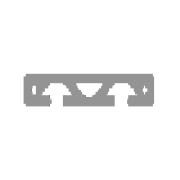
# Autodesk Inventor part: 10-081
Saved by Autodesk Inventor 2022 (Build 260153000, 153)
## iProperties
Created: 2021-12-28
Part Number: 10-081
Material: Generico
Document SubType Name: Modeling
Designer: matte
Standards Organization: 40 series
Language: it-IT
Size Designation: 10-081
Categories: <MemberInstance><Categories><Category DisplayName="Forme strutturali" InternalName="089c4875-fa83-4c05-b084-43b9cc11f5ed" Mnemonic="GRDR"><CategoryParameter DisplayName="Massa per unità di lunghezza" InternalName="0bb95a10-148f-4027-a459-38d7b056702a" Mnemonic="shpmass"/><CategoryParameter DisplayName="Area sezione" InternalName="1ff91680-64b0-4202-b9a3-7fd3f94bba3b" Mnemonic="secarea"/><CategoryParameter DisplayName="Raggio di girazione (x)" InternalName="25778675-03e9-40c1-b6a8-4a9ed693320d" Mnemonic="gyrradx"/><CategoryParameter DisplayName="Modulo di rigidità torsionale" InternalName="26c1ec35-5026-4c63-ad0a-751cf684a536" Mnemonic="torrigmod"/><CategoryParameter DisplayName="Distanza del baricentro X-X" InternalName="26c9bdb8-9c79-4b4f-a92e-8e197583c9c4" Mnemonic="grcendistX"/><CategoryParameter DisplayName="ID membro precedente" InternalName="340afe4f-75d7-48d3-ab7d-943f3c3da468" Mnemonic="LegacyMemberID"/><CategoryParameter DisplayName="Lunghezza base" InternalName="42e34263-8f20-4d0e-ad48-bf1385b87c24" Mnemonic="shplen"/><CategoryParameter DisplayName="Momento di inerzia (y)" InternalName="4b9f58ea-bced-460e-81ea-3d29ca5a49e3" Mnemonic="inermomy"/><CategoryParameter DisplayName="Momento di inerzia (x)" InternalName="4cd780bc-73d7-43ac-917a-579e5cbd684d" Mnemonic="inermomx"/><CategoryParameter DisplayName="Punto di base personalizzato" InternalName="4f1d1b73-316d-484b-a3df-9cbabb16eb77" Mnemonic="shpBasePoint"/><CategoryParameter DisplayName="Altezza forma" InternalName="50274e7d-5ac0-4796-92cb-c59e54983c67" Mnemonic="shpheig"/><CategoryParameter DisplayName="Modulo sezione (y)" InternalName="59eaa5e9-d227-48dc-b6c1-6920f96e0f95" Mnemonic="secmody"/><CategoryParameter DisplayName="Designazione sezione" InternalName="5a64d034-428d-49c8-ba32-7619764de20f" Mnemonic="shpdes"/><CategoryParameter DisplayName="Modulo sezione (x)" InternalName="72cfad18-cf51-4ed4-aaa7-c6b224f8419f" Mnemonic="secmodx"/><CategoryParameter DisplayName="Modulo di sezione torsionale" InternalName="7c55a8dc-8844-49f9-a867-cc677b30ec9a" Mnemonic="torsecmod"/><CategoryParameter DisplayName="Larghezza forma" InternalName="7c717d54-a18f-4666-b4d4-573cce22c62c" Mnemonic="shpwdth"/><CategoryParameter DisplayName="Spessore seconda forma" InternalName="9251a8e1-85fd-4e47-af99-afdb762317d9" Mnemonic="shpthick2"/><CategoryParameter DisplayName="Guarnizione piatta creata" InternalName="9c666724-f362-4ea7-ac62-f6a007de5c69" Mnemonic="shpFGAuto"/><CategoryParameter DisplayName="Distanza del baricentro Y-Y" InternalName="bcc4fb17-7af4-436a-8f8c-d0aa3b0248c5" Mnemonic="grcendistY"/><CategoryParameter DisplayName="Raggio di girazione (y)" InternalName="bfa18ebe-1636-4dbe-8d42-b263e0b73184" Mnemonic="gyrrady"/><CategoryParameter DisplayName="Spessore forma" InternalName="d109cf76-8eb4-42fc-9800-4409734adc67" Mnemonic="shpthick"/><CategoryParameter DisplayName="Coefficiente di spostamento taglio" InternalName="de4c90c6-aaa8-468f-a335-6737b311b5d3" Mnemonic="shdispc"/><Category DisplayName="Altro" InternalName="f02205ff-2390-476f-921c-0b3185f88e84" Mnemonic="OTHSHP"><CategoryParameter DisplayName="Momento di inerzia (y)" InternalName="044c654e-f649-48ac-84cc-650a29ae31ca" Mnemonic="inermomy"/><CategoryParameter DisplayName="Spessore forma" InternalName="12b1a788-9233-48fd-a933-2df8ff42b15f" Mnemonic="shpthick"/><CategoryParameter DisplayName="Massa per unità di lunghezza" InternalName="2fd289d6-9394-4d2d-97e6-6659d7d4551d" Mnemonic="shpmass"/><CategoryParameter DisplayName="Raggio di girazione (y)" InternalName="743e1dfe-1bba-408b-b985-cf752b207386" Mnemonic="gyrrady"/><CategoryParameter DisplayName="Modulo sezione (y)" InternalName="88b8bff9-a616-4028-93d5-ed4f79680d13" Mnemonic="secmody"/><CategoryParameter DisplayName="Area sezione" InternalName="c46ecdf8-b6eb-4db9-8b25-30258930c1e3" Mnemonic="secarea"/><CategoryParameter DisplayName="Modulo sezione (x)" InternalName="cac70804-9d39-43bb-be17-56ea1f39a6c2" Mnemonic="secmodx"/><CategoryParameter DisplayName="Momento di inerzia (x)" InternalName="ec6737bc-264f-43ed-b0bd-f6d410c2718d" Mnemonic="inermomx"/><CategoryParameter DisplayName="Raggio di girazione (x)" InternalName="ee72c61e-565e-4fd6-b448-66e1e1abcb7e" Mnemonic="gyrradx"/></Category></Category><Category DisplayName="TipoDati" InternalName="23b78d0f-2648-40c6-8793-ca6db495c9e8" Mnemonic="DATATYPE"><CategoryParameter DisplayName="NomeVisualizzazione" InternalName="05415f3d-3907-474b-a020-eb9d644f4cf3" Mnemonic="DISPLAYNAME"/><CategoryParameter DisplayName="Norme" InternalName="0c0a119c-1e12-4c84-803f-101930972f5e" Mnemonic="STANDARD"/><CategoryParameter DisplayName="Descrizione" InternalName="13903e3d-64b1-4950-80da-f627842ea37f" Mnemonic="DESCRIPTION"/><CategoryParameter DisplayName="Designazione" InternalName="2675968c-4ce5-49e0-a4f5-552d29089031" Mnemonic="DESIGNATION"/><CategoryParameter DisplayName="Riga di default" InternalName="2af9ec52-faaa-4026-b378-f9fa4afca842" Mnemonic="DEFAULTROW"/><CategoryParameter DisplayName="Nome cartella" InternalName="3f06958e-8713-4116-9be7-ed6184ecc97b" Mnemonic="FOLDERNAME"/><CategoryParameter DisplayName="Guid revisione" InternalName="45a75005-10b1-4dfc-8d6d-dfe629f0b93c" Mnemonic="REVISIONGUID"/><CategoryParameter DisplayName="NomeFile" InternalName="8b46a4cc-9585-4fed-90c3-899f57e09a73" Mnemonic="FILENAME"/><CategoryParameter DisplayName="SocietàNorme" InternalName="8f5914e1-4693-403f-8ab5-d37768198c9d" Mnemonic="STDSORG"/><CategoryParameter DisplayName="Versione famiglia" InternalName="914462f6-6e19-4b14-ba84-155b9680b1d0" Mnemonic="FAMILYREVISION"/><CategoryParameter DisplayName="Revisione norme" InternalName="91d5a463-65c2-4fde-b823-3b7fea5e8e17" Mnemonic="STANDARDREVISION"/><CategoryParameter DisplayName="Revisione membro" InternalName="a65d44b9-392f-4f4f-857b-e4b3d54996fe" Mnemonic="MEMBERREVISION"/><CategoryParameter DisplayName="FormatoPianoRitaglio" InternalName="bc51e27b-3422-4e78-93ef-cec197ddf230" Mnemonic="CLIPFORMAT"/><CategoryParameter DisplayName="Produttore" InternalName="cd6c7a72-a28a-4e50-99a9-2c7f4e13e5ad" Mnemonic="MANUFACTURER"/><CategoryParameter DisplayName="NomeInterno" InternalName="cf1d0246-76d9-4b4a-8305-fa0409afb5c1" Mnemonic="INTERNALNAME"/><CategoryParameter DisplayName="Èmetrico" InternalName="e2385c5b-1ea4-4823-96a8-8de651266ec3" Mnemonic="ISMETRIC"/><Category DisplayName="Parte" InternalName="c0e0b642-3bcb-4cc8-9e80-f96d35c4afa4" Mnemonic="PART"><CategoryParameter DisplayName="Numero parte" InternalName="016b6077-bfbe-49bd-92c9-d8d59c39c941" Mnemonic="PARTNUMBER"/><CategoryParameter DisplayName="Numero di magazzino" InternalName="4dba7c1c-e26c-444e-836c-b08b433409a8" Mnemonic="STOCKNUMBER"/><CategoryParameter DisplayName="Chiave materiale" InternalName="5c9a8adb-dd2b-4535-b97f-0a94a95fe41f" Mnemonic="MATERIALKEY"/><CategoryParameter DisplayName="Materiale" InternalName="818a152a-d3c3-49ca-80ee-df7d91421b8e" Mnemonic="MATERIAL"/></Category></Category></Categories><FamilyTemplate Id="10-081"><FamilyTemplateParameters><FamilyTemplateParameter ObjectType="kModelParameterObject" ValueType="xs:double" Id="12" ObjectReferenceKey="d8"/><FamilyTemplateParameter ObjectType="kPartComponentDefinitionObject" ValueType="xs:string" Id="23" SubObjectId="Material"/><FamilyTemplateParameter ObjectType="kPropertyObject" ValueType="xs:string" Id="26" ObjectReferenceKey="{32853F0F-3444-11d1-9E93-0060B03C1CA6}" SubObjectId="5"/><FamilyTemplateParameter ObjectType="kPropertyObject" ValueType="xs:string" Id="27" ObjectReferenceKey="{32853F0F-3444-11d1-9E93-0060B03C1CA6}" SubObjectId="52"/></FamilyTemplateParameters></FamilyTemplate><CategoryParameterMap><ParamToTemplateMap><ParamToTemplate CategoryParameter="//CategoryParameter[@InternalName='cf1d0246-76d9-4b4a-8305-fa0409afb5c1']" ConstantValue="b43aa390-bf45-4392-bb08-a6c8910b2740"/><ParamToTemplate CategoryParameter="//CategoryParameter[@InternalName='45a75005-10b1-4dfc-8d6d-dfe629f0b93c']" ConstantValue="b3b43e47-2cae-4de0-b985-6c6fa3d76176"/><ParamToTemplate CategoryParameter="//CategoryParameter[@InternalName='3f06958e-8713-4116-9be7-ed6184ecc97b']" ConstantValue="10-081"/><ParamToTemplate CategoryParameter="//CategoryParameter[@InternalName='8f5914e1-4693-403f-8ab5-d37768198c9d']" ConstantValue="40 series"/><ParamToTemplate CategoryParameter="//CategoryParameter[@InternalName='0c0a119c-1e12-4c84-803f-101930972f5e']" TemplateParameter="18"/><ParamToTemplate CategoryParameter="//CategoryParameter[@InternalName='91d5a463-65c2-4fde-b823-3b7fea5e8e17']" TemplateParameter="19"/><ParamToTemplate CategoryParameter="//CategoryParameter[@InternalName='cd6c7a72-a28a-4e50-99a9-2c7f4e13e5ad']" TemplateParameter="20"/><ParamToTemplate CategoryParameter="//CategoryParameter[@InternalName='13903e3d-64b1-4950-80da-f627842ea37f']" TemplateParameter="22"/><ParamToTemplate CategoryParameter="//CategoryParameter[@InternalName='05415f3d-3907-474b-a020-eb9d644f4cf3']" ConstantValue="10-081"/><ParamToTemplate CategoryParameter="//CategoryParameter[@InternalName='914462f6-6e19-4b14-ba84-155b9680b1d0']" ConstantValue="11"/><ParamToTemplate CategoryParameter="//CategoryParameter[@InternalName='bc51e27b-3422-4e78-93ef-cec197ddf230']" ConstantValue="CF_INVENTOR.STDPARTS"/><ParamToTemplate CategoryParameter="//CategoryParameter[@InternalName='e2385c5b-1ea4-4823-96a8-8de651266ec3']" ConstantValue="true"/><ParamToTemplate CategoryParameter="//CategoryParameter[@InternalName='2af9ec52-faaa-4026-b378-f9fa4afca842']" ConstantValue="1"/><ParamToTemplate CategoryParameter="//CategoryParameter[@InternalName='9c666724-f362-4ea7-ac62-f6a007de5c69']" ConstantValue="1"/><ParamToTemplate CategoryParameter="//CategoryParameter[@InternalName='8b46a4cc-9585-4fed-90c3-899f57e09a73']" ConstantValue="10-081"/><ParamToTemplate CategoryParameter="//CategoryParameter[@InternalName='a65d44b9-392f-4f4f-857b-e4b3d54996fe']" ConstantValue="bb38fb4f-2023-4888-b702-42cbc433ea70"/><ParamToTemplate CategoryParameter="//CategoryParameter[@InternalName='a65d44b9-392f-4f4f-857b-e4b3d54996fe']" ConstantValue="bb38fb4f-2023-4888-b702-42cbc433ea70"/><ParamToTemplate CategoryParameter="//CategoryParameter[@InternalName='2675968c-4ce5-49e0-a4f5-552d29089031']" TemplateParameter="27"/><ParamToTemplate CategoryParameter="//CategoryParameter[@InternalName='818a152a-d3c3-49ca-80ee-df7d91421b8e']" TemplateParameter="23"/><ParamToTemplate CategoryParameter="//CategoryParameter[@InternalName='016b6077-bfbe-49bd-92c9-d8d59c39c941']" TemplateParameter="26"/><ParamToTemplate CategoryParameter="//CategoryParameter[@InternalName='42e34263-8f20-4d0e-ad48-bf1385b87c24']" TemplateParameter="12"/></ParamToTemplateMap></CategoryParameterMap></MemberInstance>
Density: 1 g/cm^3
Appearance: Default
MXEDIT: true
G_L: 240,000 mm
IsCustomPart: 1
Author: matte
Autodesk Inventor part; units mm, degrees
ref_plane "YZ Plane" through (0, 0, 0) normal (1, 0, 0) x (0, 1, 0)
ref_plane "Start Plane" through (0, 0, 0) normal (0, 1, 0) x (-1, 0, 0)
ref_plane "End Plane" through (0, 240, 0) normal (0, 1, 0) x (-1, 0, 0)
sketch "Sketch1" plane through (0, 0, 0) normal (0, 1, 0) x (-1, 0, 0)
  line L0 (40, -5) -> (40, 5)
  arc A0 (40, 5) -> (37, 8) centre (37, 5) ccw
  line L1 (37, 8) -> (-37, 8)
  line L2 (14.5, -8) -> (-14.5, -8)
  arc A1 (14.5, -8) -> (16, -6.5) centre (14.5, -6.5) ccw
  line L3 (-25.5, -8) -> (-37, -8)
  arc A2 (-25.5, -8) -> (-24, -6.5) centre (-25.5, -6.5) ccw
  arc A3 (-37, 8) -> (-40, 5) centre (-37, 5) ccw
  line L4 (-40, 5) -> (-40, -5)
  arc A4 (-40, -5) -> (-37, -8) centre (-37, -5) ccw
  line L5 (-24, -6.5) -> (-24, -4.5)
  arc A5 (-24, -4.5) -> (-25, -3.5) centre (-25, -4.5) ccw
  line L6 (-25, -3.5) -> (-29.0014, -3.5)
  arc A6 (-29.8106, -1.9125) -> (-29.0014, -3.5) centre (-29.0014, -2.5) ccw
  arc A7 (-23.7664, 3.9851) -> (-29.8106, -1.9125) centre (-9.58, -16.6) ccw
  arc A8 (-22.9152, 4.25) -> (-23.7664, 3.9851) centre (-22.9152, 2.75) ccw
  line L7 (-22.9152, 4.25) -> (-17.0848, 4.25)
  arc A9 (-16.2336, 3.9851) -> (-17.0848, 4.25) centre (-17.0848, 2.75) ccw
  arc A10 (-10.1894, -1.9125) -> (-16.2336, 3.9851) centre (-30.42, -16.6) ccw
  arc A11 (-10.9986, -3.5) -> (-10.1894, -1.9125) centre (-10.9986, -2.5) ccw
  line L8 (-10.9986, -3.5) -> (-15, -3.5)
  arc A12 (-15, -3.5) -> (-16, -4.5) centre (-15, -4.5) ccw
  line L9 (-16, -4.5) -> (-16, -6.5)
  arc A13 (-16, -6.5) -> (-14.5, -8) centre (-14.5, -6.5) ccw
  line L10 (16, -6.5) -> (16, -4.5)
  arc A14 (16, -4.5) -> (15, -3.5) centre (15, -4.5) ccw
  line L11 (15, -3.5) -> (10.9986, -3.5)
  arc A15 (10.1894, -1.9125) -> (10.9986, -3.5) centre (10.9986, -2.5) ccw
  arc A16 (16.2336, 3.9851) -> (10.1894, -1.9125) centre (30.42, -16.6) ccw
  arc A17 (17.0848, 4.25) -> (16.2336, 3.9851) centre (17.0848, 2.75) ccw
  line L12 (17.0848, 4.25) -> (22.9152, 4.25)
  arc A18 (23.7664, 3.9851) -> (22.9152, 4.25) centre (22.9152, 2.75) ccw
  arc A19 (29.8106, -1.9125) -> (23.7664, 3.9851) centre (9.58, -16.6) ccw
  arc A20 (29.0014, -3.5) -> (29.8106, -1.9125) centre (29.0014, -2.5) ccw
  line L13 (29.0014, -3.5) -> (25, -3.5)
  arc A21 (25, -3.5) -> (24, -4.5) centre (25, -4.5) ccw
  line L14 (1.9858, -3.8) -> (-1.9858, -3.8)
  arc A22 (-2.6929, -3.5071) -> (-1.9858, -3.8) centre (-1.9858, -2.8) ccw
  line L15 (-2.6929, -3.5071) -> (-8.2929, 2.0929)
  arc A23 (-7.5858, 3.8) -> (-8.2929, 2.0929) centre (-7.5858, 2.8) ccw
  line L16 (-7.5858, 3.8) -> (7.5858, 3.8)
  arc A24 (8.2929, 2.0929) -> (7.5858, 3.8) centre (7.5858, 2.8) ccw
  line L17 (8.2929, 2.0929) -> (2.6929, -3.5071)
  arc A25 (1.9858, -3.8) -> (2.6929, -3.5071) centre (1.9858, -2.8) ccw
  circle A26 centre (-34, 0) radius 2.05
  circle A27 centre (34, 0) radius 2.05
  line L18 (25.5, -8) -> (37, -8)
  arc A28 (24, -6.5) -> (25.5, -8) centre (25.5, -6.5) ccw
  arc A29 (37, -8) -> (40, -5) centre (37, -5) ccw
  line L19 (24, -6.5) -> (24, -4.5)
  point P0 (0, 0)
  constraints: 56 point on circle, 40 end point, 30 centre point, 12 horizontal, 6 vertical, 111 other
extrude "Body" add sketch "Sketch1" along normal up to surface (240 mm away) from surface at 0
sketch "Sketch2" plane through (0, 0, 0) normal (0, 1, 0) x (-1, 0, 0)
  line L0 (0, 0) -> (10, 0)
ref_plane "Work Plane3" through (0, 0, 0) normal (0, 0, -1) x (-1, 0, 0)
sketch "Sketch3" plane through (0, 0, 0) normal (0, 0, -1) x (-1, 0, 0)
  line L0 (-2, 0) -> (12, 0)
  line L1 (-2, 240) -> (12, 240)
  dimension "d15" = 240
  measures "d15" distance between parallel lines of L0 L1
sketch "Schizzo4" plane through (22.9152, 240, 4.25) normal (0, 0, -1) x (-1, 0, 0)
  point P0 (22.9152, -240)
equation "\"G_OFFSET_START\" = 0"
equation "\"G_OFFSET_END\" = 0"
equation "\"G_L\" = d15"
body "Solid1"
